Autodesk Inventor part; units mm, degrees
(part 2 of 2)
  spline S181 degree 2 poles (82.302, -43.6262) (81.9786, -43.6262) (81.5787, -43.9297) (81.5787, -44.1764) knots 0 0 0 1 2 2 2
  spline S182 degree 2 poles (81.5787, -44.1764) (81.5787, -44.3977) (81.8141, -44.6614) (82.0353, -44.721) knots 0 0 0 1 2 2 2
  spline S183 degree 2 poles (82.0353, -44.721) (82.1828, -44.7607) (82.6111, -44.8628) (82.7529, -44.9054) knots 0 0 0 1 2 2 2
  spline S184 degree 2 poles (82.7529, -44.9054) (83.1131, -45.016) (83.4478, -45.4613) (83.4478, -45.7875) knots 0 0 0 1 2 2 2
  spline S185 degree 2 poles (83.4478, -45.7875) (83.4478, -45.9945) (83.2805, -46.3916) (83.1302, -46.5306) knots 0 0 0 1 2 2 2
  spline S186 degree 2 poles (83.1302, -46.5306) (82.9628, -46.6837) (82.5374, -46.8482) (82.2169, -46.8482) knots 0 0 0 1 2 2 2
  line L442 (86.3721, -43.2858) -> (85.1893, -45.2372)
  line L443 (85.1893, -45.2372) -> (85.1893, -46.7858)
  line L444 (85.1893, -46.7858) -> (84.7242, -46.7858)
  line L445 (84.7242, -46.7858) -> (84.7242, -45.2854)
  line L446 (84.7242, -45.2854) -> (83.5414, -43.2858)
  line L447 (83.5414, -43.2858) -> (84.0576, -43.2858)
  line L448 (84.0576, -43.2858) -> (84.9596, -44.826)
  line L449 (84.9596, -44.826) -> (85.8785, -43.2858)
  line L450 (85.8785, -43.2858) -> (86.3721, -43.2858)
  spline S187 degree 2 poles (87.6711, -46.8482) (87.291, -46.8482) (86.7578, -46.6894) (86.5224, -46.576) knots 0 0 0 1 2 2 2
  line L451 (86.5224, -46.576) -> (86.5224, -45.9917)
  line L452 (86.5224, -45.9917) -> (86.5564, -45.9917)
  spline S188 degree 2 poles (86.5564, -45.9917) (86.7862, -46.2072) (87.3676, -46.4455) (87.637, -46.4455) knots 0 0 0 1 2 2 2
  spline S189 degree 2 poles (87.637, -46.4455) (88.0228, -46.4455) (88.417, -46.125) (88.417, -45.8612) knots 0 0 0 1 2 2 2
  spline S190 degree 2 poles (88.417, -45.8612) (88.417, -45.6513) (88.21, -45.3904) (87.9859, -45.3251) knots 0 0 0 1 2 2 2
  spline S191 degree 2 poles (87.9859, -45.3251) (87.8242, -45.2798) (87.5548, -45.2174) (87.3534, -45.1663) knots 0 0 0 1 2 2 2
  spline S192 degree 2 poles (87.3534, -45.1663) (87.1719, -45.1181) (86.8854, -44.9734) (86.7748, -44.8572) knots 0 0 0 1 2 2 2
  spline S193 degree 2 poles (86.7748, -44.8572) (86.667, -44.7409) (86.5479, -44.4289) (86.5479, -44.2247) knots 0 0 0 1 2 2 2
  spline S194 degree 2 poles (86.5479, -44.2247) (86.5479, -43.7992) (87.2116, -43.2234) (87.725, -43.2234) knots 0 0 0 1 2 2 2
  spline S195 degree 2 poles (87.725, -43.2234) (88.0199, -43.2234) (88.5418, -43.3397) (88.7659, -43.4503) knots 0 0 0 1 2 2 2
  line L453 (88.7659, -43.4503) -> (88.7659, -44.0063)
  line L454 (88.7659, -44.0063) -> (88.7319, -44.0063)
  spline S196 degree 2 poles (88.7319, -44.0063) (88.5645, -43.8531) (88.0426, -43.6262) (87.7562, -43.6262) knots 0 0 0 1 2 2 2
  spline S197 degree 2 poles (87.7562, -43.6262) (87.4328, -43.6262) (87.0329, -43.9297) (87.0329, -44.1764) knots 0 0 0 1 2 2 2
  spline S198 degree 2 poles (87.0329, -44.1764) (87.0329, -44.3977) (87.2683, -44.6614) (87.4896, -44.721) knots 0 0 0 1 2 2 2
  spline S199 degree 2 poles (87.4896, -44.721) (87.637, -44.7607) (88.0653, -44.8628) (88.2071, -44.9054) knots 0 0 0 1 2 2 2
  spline S200 degree 2 poles (88.2071, -44.9054) (88.5674, -45.016) (88.902, -45.4613) (88.902, -45.7875) knots 0 0 0 1 2 2 2
  spline S201 degree 2 poles (88.902, -45.7875) (88.902, -45.9945) (88.7347, -46.3916) (88.5844, -46.5306) knots 0 0 0 1 2 2 2
  spline S202 degree 2 poles (88.5844, -46.5306) (88.417, -46.6837) (87.9916, -46.8482) (87.6711, -46.8482) knots 0 0 0 1 2 2 2
  line L455 (90.1926, -46.7858) -> (90.1926, -43.6999)
  line L456 (90.1926, -43.6999) -> (89.0183, -43.6999)
  line L457 (89.0183, -43.6999) -> (89.0183, -43.2858)
  line L458 (89.0183, -43.2858) -> (91.8319, -43.2858)
  line L459 (91.8319, -43.2858) -> (91.8319, -43.6999)
  line L460 (91.8319, -43.6999) -> (90.6577, -43.6999)
  line L461 (90.6577, -43.6999) -> (90.6577, -46.7858)
  line L462 (90.6577, -46.7858) -> (90.1926, -46.7858)
  line L463 (92.1865, -46.7858) -> (92.1865, -43.2858)
  line L464 (92.1865, -43.2858) -> (94.3761, -43.2858)
  line L465 (94.3761, -43.2858) -> (94.3761, -43.6999)
  line L466 (94.3761, -43.6999) -> (92.6516, -43.6999)
  line L467 (92.6516, -43.6999) -> (92.6516, -44.6586)
  line L468 (92.6516, -44.6586) -> (94.2598, -44.6586)
  line L469 (94.2598, -44.6586) -> (94.2598, -45.0727)
  line L470 (94.2598, -45.0727) -> (92.6516, -45.0727)
  line L471 (92.6516, -45.0727) -> (92.6516, -46.3717)
  line L472 (92.6516, -46.3717) -> (94.3761, -46.3717)
  line L473 (94.3761, -46.3717) -> (94.3761, -46.7858)
  line L474 (94.3761, -46.7858) -> (92.1865, -46.7858)
  line L475 (97.8875, -46.7858) -> (97.4223, -46.7858)
  line L476 (97.4223, -46.7858) -> (97.4223, -43.7708)
  line L477 (97.4223, -43.7708) -> (96.509, -45.8215)
  line L478 (96.509, -45.8215) -> (96.2254, -45.8215)
  line L479 (96.2254, -45.8215) -> (95.3206, -43.7708)
  line L480 (95.3206, -43.7708) -> (95.3206, -46.7858)
  line L481 (95.3206, -46.7858) -> (94.8866, -46.7858)
  line L482 (94.8866, -46.7858) -> (94.8866, -43.2858)
  line L483 (94.8866, -43.2858) -> (95.522, -43.2858)
  line L484 (95.522, -43.2858) -> (96.3956, -45.2344)
  line L485 (96.3956, -45.2344) -> (97.2408, -43.2858)
  line L486 (97.2408, -43.2858) -> (97.8875, -43.2858)
  line L487 (97.8875, -43.2858) -> (97.8875, -46.7858)
  line L488 (51.2813, -51.3459) -> (50.8644, -51.3459)
  line L489 (50.8644, -51.3459) -> (50.8644, -52.5485)
  line L490 (50.8644, -52.5485) -> (50.4134, -52.5485)
  line L491 (50.4134, -52.5485) -> (50.4134, -51.3459)
  line L492 (50.4134, -51.3459) -> (48.8676, -51.3459)
  line L493 (48.8676, -51.3459) -> (48.8676, -50.8524)
  line L494 (48.8676, -50.8524) -> (50.4332, -49.0485)
  line L495 (50.4332, -49.0485) -> (50.8644, -49.0485)
  line L496 (50.8644, -49.0485) -> (50.8644, -50.9687)
  line L497 (50.8644, -50.9687) -> (51.2813, -50.9687)
  line L498 (51.2813, -50.9687) -> (51.2813, -51.3459)
  line L499 (50.4134, -50.9687) -> (50.4134, -49.6016)
  line L500 (50.4134, -49.6016) -> (49.2363, -50.9687)
  line L501 (49.2363, -50.9687) -> (50.4134, -50.9687)
  spline S203 degree 2 poles (52.6002, -49.3803) (52.4725, -49.3803) (52.2201, -49.4427) (52.0981, -49.491) knots 0 0 0 1 2 2 2
  spline S204 degree 2 poles (52.0981, -49.491) (51.9847, -49.5392) (51.8174, -49.6413) (51.7521, -49.6867) knots 0 0 0 1 2 2 2
  line L502 (51.7521, -49.6867) -> (51.7238, -49.6867)
  line L503 (51.7238, -49.6867) -> (51.7238, -49.1903)
  spline S205 degree 2 poles (51.7238, -49.1903) (51.8769, -49.1081) (52.4016, -48.9748) (52.637, -48.9748) knots 0 0 0 1 2 2 2
  spline S206 degree 2 poles (52.637, -48.9748) (52.8753, -48.9748) (53.2298, -49.0712) (53.3745, -49.1733) knots 0 0 0 1 2 2 2
  spline S207 degree 2 poles (53.3745, -49.1733) (53.5276, -49.2839) (53.6865, -49.6044) (53.6865, -49.82) knots 0 0 0 1 2 2 2
  spline S208 degree 2 poles (53.6865, -49.82) (53.6865, -50.1093) (53.3064, -50.5461) (53.0398, -50.6028) knots 0 0 0 1 2 2 2
  line L504 (53.0398, -50.6028) -> (53.0398, -50.6368)
  spline S209 degree 2 poles (53.0398, -50.6368) (53.1504, -50.6595) (53.4028, -50.7616) (53.5106, -50.8637) knots 0 0 0 1 2 2 2
  spline S210 degree 2 poles (53.5106, -50.8637) (53.6184, -50.963) (53.7546, -51.2807) (53.7546, -51.5104) knots 0 0 0 1 2 2 2
  spline S211 degree 2 poles (53.7546, -51.5104) (53.7546, -51.7458) (53.5929, -52.1457) (53.4454, -52.2989) knots 0 0 0 1 2 2 2
  spline S212 degree 2 poles (53.4454, -52.2989) (53.2922, -52.4577) (52.8583, -52.6222) (52.5832, -52.6222) knots 0 0 0 1 2 2 2
  spline S213 degree 2 poles (52.5832, -52.6222) (52.3194, -52.6222) (51.8032, -52.4946) (51.6273, -52.4067) knots 0 0 0 1 2 2 2
  line L505 (51.6273, -52.4067) -> (51.6273, -51.9103)
  line L506 (51.6273, -51.9103) -> (51.6614, -51.9103)
  spline S214 degree 2 poles (51.6614, -51.9103) (51.8088, -52.0181) (52.308, -52.2167) (52.5548, -52.2167) knots 0 0 0 1 2 2 2
  spline S215 degree 2 poles (52.5548, -52.2167) (52.6994, -52.2167) (52.9887, -52.1259) (53.0852, -52.0209) knots 0 0 0 1 2 2 2
  spline S216 degree 2 poles (53.0852, -52.0209) (53.1788, -51.916) (53.2781, -51.6664) (53.2781, -51.4764) knots 0 0 0 1 2 2 2
  spline S217 degree 2 poles (53.2781, -51.4764) (53.2781, -51.2863) (53.1674, -51.0396) (53.0682, -50.9687) knots 0 0 0 1 2 2 2
  spline S218 degree 2 poles (53.0682, -50.9687) (52.9689, -50.8978) (52.6994, -50.8439) (52.5406, -50.8439) knots 0 0 0 1 2 2 2
  line L507 (52.5406, -50.8439) -> (52.3421, -50.8439)
  line L508 (52.3421, -50.8439) -> (52.3421, -50.4553)
  line L509 (52.3421, -50.4553) -> (52.4981, -50.4553)
  spline S219 degree 2 poles (52.4981, -50.4553) (52.8129, -50.4553) (53.21, -50.1547) (53.21, -49.8682) knots 0 0 0 1 2 2 2
  spline S220 degree 2 poles (53.21, -49.8682) (53.21, -49.7349) (53.1079, -49.5449) (53.0256, -49.4881) knots 0 0 0 1 2 2 2
  spline S221 degree 2 poles (53.0256, -49.4881) (52.9377, -49.4286) (52.7221, -49.3803) (52.6002, -49.3803) knots 0 0 0 1 2 2 2
  spline S222 degree 2 poles (55.2266, -49.3803) (55.099, -49.3803) (54.8465, -49.4427) (54.7246, -49.491) knots 0 0 0 1 2 2 2
  spline S223 degree 2 poles (54.7246, -49.491) (54.6111, -49.5392) (54.4438, -49.6413) (54.3785, -49.6867) knots 0 0 0 1 2 2 2
  line L510 (54.3785, -49.6867) -> (54.3502, -49.6867)
  line L511 (54.3502, -49.6867) -> (54.3502, -49.1903)
  spline S224 degree 2 poles (54.3502, -49.1903) (54.5033, -49.1081) (55.0281, -48.9748) (55.2635, -48.9748) knots 0 0 0 1 2 2 2
  spline S225 degree 2 poles (55.2635, -48.9748) (55.5017, -48.9748) (55.8563, -49.0712) (56.0009, -49.1733) knots 0 0 0 1 2 2 2
  spline S226 degree 2 poles (56.0009, -49.1733) (56.1541, -49.2839) (56.3129, -49.6044) (56.3129, -49.82) knots 0 0 0 1 2 2 2
  spline S227 degree 2 poles (56.3129, -49.82) (56.3129, -50.1093) (55.9328, -50.5461) (55.6662, -50.6028) knots 0 0 0 1 2 2 2
  line L512 (55.6662, -50.6028) -> (55.6662, -50.6368)
  spline S228 degree 2 poles (55.6662, -50.6368) (55.7768, -50.6595) (56.0293, -50.7616) (56.137, -50.8637) knots 0 0 0 1 2 2 2
  spline S229 degree 2 poles (56.137, -50.8637) (56.2448, -50.963) (56.381, -51.2807) (56.381, -51.5104) knots 0 0 0 1 2 2 2
  spline S230 degree 2 poles (56.381, -51.5104) (56.381, -51.7458) (56.2193, -52.1457) (56.0718, -52.2989) knots 0 0 0 1 2 2 2
  spline S231 degree 2 poles (56.0718, -52.2989) (55.9187, -52.4577) (55.4847, -52.6222) (55.2096, -52.6222) knots 0 0 0 1 2 2 2
  spline S232 degree 2 poles (55.2096, -52.6222) (54.9458, -52.6222) (54.4296, -52.4946) (54.2537, -52.4067) knots 0 0 0 1 2 2 2
  line L513 (54.2537, -52.4067) -> (54.2537, -51.9103)
  line L514 (54.2537, -51.9103) -> (54.2878, -51.9103)
  spline S233 degree 2 poles (54.2878, -51.9103) (54.4353, -52.0181) (54.9345, -52.2167) (55.1812, -52.2167) knots 0 0 0 1 2 2 2
  spline S234 degree 2 poles (55.1812, -52.2167) (55.3259, -52.2167) (55.6152, -52.1259) (55.7116, -52.0209) knots 0 0 0 1 2 2 2
  spline S235 degree 2 poles (55.7116, -52.0209) (55.8052, -51.916) (55.9045, -51.6664) (55.9045, -51.4764) knots 0 0 0 1 2 2 2
  spline S236 degree 2 poles (55.9045, -51.4764) (55.9045, -51.2863) (55.7939, -51.0396) (55.6946, -50.9687) knots 0 0 0 1 2 2 2
  spline S237 degree 2 poles (55.6946, -50.9687) (55.5953, -50.8978) (55.3259, -50.8439) (55.167, -50.8439) knots 0 0 0 1 2 2 2
  line L515 (55.167, -50.8439) -> (54.9685, -50.8439)
  line L516 (54.9685, -50.8439) -> (54.9685, -50.4553)
  line L517 (54.9685, -50.4553) -> (55.1245, -50.4553)
  spline S238 degree 2 poles (55.1245, -50.4553) (55.4393, -50.4553) (55.8364, -50.1547) (55.8364, -49.8682) knots 0 0 0 1 2 2 2
  spline S239 degree 2 poles (55.8364, -49.8682) (55.8364, -49.7349) (55.7343, -49.5449) (55.652, -49.4881) knots 0 0 0 1 2 2 2
  spline S240 degree 2 poles (55.652, -49.4881) (55.5641, -49.4286) (55.3486, -49.3803) (55.2266, -49.3803) knots 0 0 0 1 2 2 2
  line L518 (60.0086, -52.5485) -> (59.5434, -52.5485)
  line L519 (59.5434, -52.5485) -> (59.5434, -49.5335)
  line L520 (59.5434, -49.5335) -> (58.6302, -51.5842)
  line L521 (58.6302, -51.5842) -> (58.3465, -51.5842)
  line L522 (58.3465, -51.5842) -> (57.4417, -49.5335)
  line L523 (57.4417, -49.5335) -> (57.4417, -52.5485)
  line L524 (57.4417, -52.5485) -> (57.0078, -52.5485)
  line L525 (57.0078, -52.5485) -> (57.0078, -49.0485)
  line L526 (57.0078, -49.0485) -> (57.6431, -49.0485)
  line L527 (57.6431, -49.0485) -> (58.5167, -50.997)
  line L528 (58.5167, -50.997) -> (59.3619, -49.0485)
  line L529 (59.3619, -49.0485) -> (60.0086, -49.0485)
  line L530 (60.0086, -49.0485) -> (60.0086, -52.5485)
  line L531 (63.259, -52.5485) -> (62.7939, -52.5485)
  line L532 (62.7939, -52.5485) -> (62.7939, -50.8354)
  line L533 (62.7939, -50.8354) -> (61.1828, -50.8354)
  line L534 (61.1828, -50.8354) -> (61.1828, -52.5485)
  line L535 (61.1828, -52.5485) -> (60.7177, -52.5485)
  line L536 (60.7177, -52.5485) -> (60.7177, -49.0485)
  line L537 (60.7177, -49.0485) -> (61.1828, -49.0485)
  line L538 (61.1828, -49.0485) -> (61.1828, -50.4213)
  line L539 (61.1828, -50.4213) -> (62.7939, -50.4213)
  line L540 (62.7939, -50.4213) -> (62.7939, -49.0485)
  line L541 (62.7939, -49.0485) -> (63.259, -49.0485)
  line L542 (63.259, -49.0485) -> (63.259, -52.5485)
  line L543 (66.2003, -52.5485) -> (63.7554, -52.5485)
  line L544 (63.7554, -52.5485) -> (63.7554, -52.1145)
  line L545 (63.7554, -52.1145) -> (65.6273, -49.4626)
  line L546 (65.6273, -49.4626) -> (63.8404, -49.4626)
  line L547 (63.8404, -49.4626) -> (63.8404, -49.0485)
  line L548 (63.8404, -49.0485) -> (66.152, -49.0485)
  line L549 (66.152, -49.0485) -> (66.152, -49.4683)
  line L550 (66.152, -49.4683) -> (64.2602, -52.1344)
  line L551 (64.2602, -52.1344) -> (66.2003, -52.1344)
  line L552 (66.2003, -52.1344) -> (66.2003, -52.5485)
  line L553 (69.3826, -52.5485) -> (68.0268, -52.5485)
  line L554 (68.0268, -52.5485) -> (68.0268, -52.1911)
  line L555 (68.0268, -52.1911) -> (68.4721, -52.1911)
  line L556 (68.4721, -52.1911) -> (68.4721, -49.4059)
  line L557 (68.4721, -49.4059) -> (68.0268, -49.4059)
  line L558 (68.0268, -49.4059) -> (68.0268, -49.0485)
  line L559 (68.0268, -49.0485) -> (69.3826, -49.0485)
  line L560 (69.3826, -49.0485) -> (69.3826, -49.4059)
  line L561 (69.3826, -49.4059) -> (68.9373, -49.4059)
  line L562 (68.9373, -49.4059) -> (68.9373, -52.1911)
  line L563 (68.9373, -52.1911) -> (69.3826, -52.1911)
  line L564 (69.3826, -52.1911) -> (69.3826, -52.5485)
  spline S241 degree 2 poles (70.934, -52.6109) (70.554, -52.6109) (70.0208, -52.4521) (69.7853, -52.3386) knots 0 0 0 1 2 2 2
  line L565 (69.7853, -52.3386) -> (69.7853, -51.7543)
  line L566 (69.7853, -51.7543) -> (69.8194, -51.7543)
  spline S242 degree 2 poles (69.8194, -51.7543) (70.0491, -51.9699) (70.6306, -52.2081) (70.9, -52.2081) knots 0 0 0 1 2 2 2
  spline S243 degree 2 poles (70.9, -52.2081) (71.2857, -52.2081) (71.68, -51.8876) (71.68, -51.6239) knots 0 0 0 1 2 2 2
  spline S244 degree 2 poles (71.68, -51.6239) (71.68, -51.414) (71.4729, -51.153) (71.2489, -51.0878) knots 0 0 0 1 2 2 2
  spline S245 degree 2 poles (71.2489, -51.0878) (71.0872, -51.0424) (70.8178, -50.98) (70.6164, -50.929) knots 0 0 0 1 2 2 2
  spline S246 degree 2 poles (70.6164, -50.929) (70.4349, -50.8808) (70.1484, -50.7361) (70.0378, -50.6198) knots 0 0 0 1 2 2 2
  spline S247 degree 2 poles (70.0378, -50.6198) (69.93, -50.5035) (69.8109, -50.1915) (69.8109, -49.9873) knots 0 0 0 1 2 2 2
  spline S248 degree 2 poles (69.8109, -49.9873) (69.8109, -49.5619) (70.4746, -48.9861) (70.9879, -48.9861) knots 0 0 0 1 2 2 2
  spline S249 degree 2 poles (70.9879, -48.9861) (71.2829, -48.9861) (71.8048, -49.1024) (72.0289, -49.213) knots 0 0 0 1 2 2 2
  line L567 (72.0289, -49.213) -> (72.0289, -49.7689)
  line L568 (72.0289, -49.7689) -> (71.9948, -49.7689)
  spline S250 degree 2 poles (71.9948, -49.7689) (71.8275, -49.6158) (71.3056, -49.3889) (71.0191, -49.3889) knots 0 0 0 1 2 2 2
  spline S251 degree 2 poles (71.0191, -49.3889) (70.6958, -49.3889) (70.2959, -49.6923) (70.2959, -49.9391) knots 0 0 0 1 2 2 2
  spline S252 degree 2 poles (70.2959, -49.9391) (70.2959, -50.1603) (70.5313, -50.4241) (70.7525, -50.4837) knots 0 0 0 1 2 2 2
  spline S253 degree 2 poles (70.7525, -50.4837) (70.9, -50.5234) (71.3283, -50.6255) (71.4701, -50.668) knots 0 0 0 1 2 2 2
  spline S254 degree 2 poles (71.4701, -50.668) (71.8303, -50.7786) (72.165, -51.2239) (72.165, -51.5501) knots 0 0 0 1 2 2 2
  spline S255 degree 2 poles (72.165, -51.5501) (72.165, -51.7572) (71.9977, -52.1543) (71.8473, -52.2932) knots 0 0 0 1 2 2 2
  spline S256 degree 2 poles (71.8473, -52.2932) (71.68, -52.4464) (71.2546, -52.6109) (70.934, -52.6109) knots 0 0 0 1 2 2 2
  line L569 (75.6395, -52.5485) -> (75.1743, -52.5485)
  line L570 (75.1743, -52.5485) -> (75.1743, -49.5335)
  line L571 (75.1743, -49.5335) -> (74.261, -51.5842)
  line L572 (74.261, -51.5842) -> (73.9774, -51.5842)
  line L573 (73.9774, -51.5842) -> (73.0726, -49.5335)
  line L574 (73.0726, -49.5335) -> (73.0726, -52.5485)
  line L575 (73.0726, -52.5485) -> (72.6387, -52.5485)
  line L576 (72.6387, -52.5485) -> (72.6387, -49.0485)
  line L577 (72.6387, -49.0485) -> (73.274, -49.0485)
  line L578 (73.274, -49.0485) -> (74.1476, -50.997)
  line L579 (74.1476, -50.997) -> (74.9928, -49.0485)
  line L580 (74.9928, -49.0485) -> (75.6395, -49.0485)
  line L581 (75.6395, -49.0485) -> (75.6395, -52.5485)
  point P0 (0, 0)
  constraints: 2 other
emboss "Emboss1" sketch "Sketch4" operation cut depth 1 direction (0, 1, 0)
body "Solid1"
